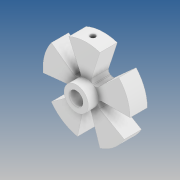
# Autodesk Inventor part: 1313_Drive Coil End_V1
Saved by Autodesk Inventor 2020 (Build 240168000, 168)
## iProperties
Created: 2019-10-22
Part Number: 1313_Drive Coil End_V1
Material: ABS Plastic
Document SubType Name: Modeling
Designer: RFLab
Density: 1.06 g/cm^3
Appearance: Smooth - White
Author: RFLab
Autodesk Inventor part; units mm, degrees
ref_plane "YZ Plane" through (0, 0, 0) normal (1, 0, 0) x (0, 1, 0)
ref_plane "XZ Plane" through (0, 0, 0) normal (0, 1, 0) x (-1, 0, 0)
sketch "Sketch1" plane through (0, 0, 0) normal (0, 0, 1) x (1, 0, 0)
  circle A0 centre (0, 0) radius 25.2
  dimension "d0" = 50.4
  constraints: 1 centre point, 1 coincident
  measures "d0" diameter of A0
sketch "Sketch1 outline for Extrusion1" plane through (0, 0, 0) normal (0, 0, 1) x (1, 0, 0)
  circle A0 centre (0, 0) radius 25.2
extrude "Extrusion1" add sketch "Sketch1 outline for Extrusion1" along normal blind 10
sketch "Sketch2" plane through (0, 0, 10) normal (0, 0, 1) x (1, 0, 0)
  circle A0 centre (0, 0) radius 25.2 projected
  circle A1 centre (0, 0) radius 7
  dimension "d3" = 14
  constraints: 1 centre point, 1 coincident
  measures "d3" diameter of A1
sketch "Sketch2 outline for Extrusion2" plane through (0, 0, 10) normal (0, 0, 1) x (1, 0, 0)
  circle A0 centre (0, 0) radius 7
extrude "Extrusion2" add sketch "Sketch2 outline for Extrusion2" along normal blind 6
sketch "Sketch4" plane through (0, 0, 16) normal (0, 0, 1) x (1, 0, 0)
  circle A0 centre (0, 0) radius 7 projected
  circle A1 centre (0, 0) radius 4
  dimension "d9" = 8
  constraints: 1 centre point, 1 coincident
  measures "d9" diameter of A1
sketch "Sketch4 outline for Extrusion4" plane through (0, 0, 16) normal (0, 0, 1) x (1, 0, 0)
  circle A0 centre (0, 0) radius 4
extrude "Extrusion4" cut sketch "Sketch4 outline for Extrusion4" against normal through all
sketch "Sketch8" plane through (0, 0, 0) normal (0, 0, -1) x (-1, 0, 0)
  line L0 (0, 0) -> (-25.2, 0)
  circle A0 centre (0, 0) radius 25.2
  circle A1 centre (0, 0) radius 7
  line L1 (0, 0) -> (-21.82384, -12.6)
  point P0 (-6.062178, -3.5)
  point P1 (-7, 0)
  dimension "d23" = 30
  constraints: 4 end point, 2 point on circle, 1 horizontal
  measures "d23" angle of L1 L0
sketch "Sketch8 outline for Extrusion8" plane through (0, 0, 0) normal (0, 0, -1) x (-1, 0, 0)
  line L0 (-21.82384, -12.6) -> (-6.062178, -3.5)
  arc A0 (-25.2, 0) -> (-21.82384, -12.6) centre (0, 0) ccw
  line L1 (-7, 0) -> (-25.2, 0)
  arc A1 (-6.062178, -3.5) -> (-7, 0) centre (0, 0) cw
extrude "Extrusion8" cut sketch "Sketch8 outline for Extrusion8" against normal blind 10
pattern_circular "Circular Pattern1" count 5 over 360 about axis through (0, 0, 16) along (0, 0, -1) of "Extrusion8"
fillet "Fillet1" radius 2 10 edges at (5.202, 4.6839, 5) (2.1631, 6.6574, 5) (-2.8472, 6.3948, 5) (-5.6631, 4.1145, 5) (-6.9617, -0.7317, 5) (-5.6631, -4.1145, 5) (-1.4554, -6.847, 5) (2.1631, -6.6574, 5) (7, 0, 5) (6.0622, -3.5, 5)
ref_plane "Work Plane1" through (-1.318866, 25.165464, 0) normal (-0.052336, 0.9986295, 0) x (-0.9986295, -0.052336, 0)
sketch "Sketch9" plane through (-1.318866, 25.165464, 0) normal (-0.052336, 0.9986295, 0) x (-0.9986295, -0.052336, 0)
  circle A0 centre (0, 5) radius 1.5
  point P0 (0, 0)
  dimension "d30" = 3
  dimension "d31" = 5
  constraints: 1 centre point
  measures "d30" diameter of A0
  measures "d31" distance of point (0, 0) A0.centre
sketch "Sketch9 outline for Extrusion9" plane through (-1.318866, 25.165464, 0) normal (-0.052336, 0.9986295, 0) x (-0.9986295, -0.052336, 0)
  circle A0 centre (0, 5) radius 1.5
extrude "Extrusion9" cut sketch "Sketch9 outline for Extrusion9" against normal blind 5
pattern_circular "Circular Pattern2" count 2 over 144 about axis through (0, 0, 16) along (0, 0, 1) of "Extrusion9"
body "Solid1"
